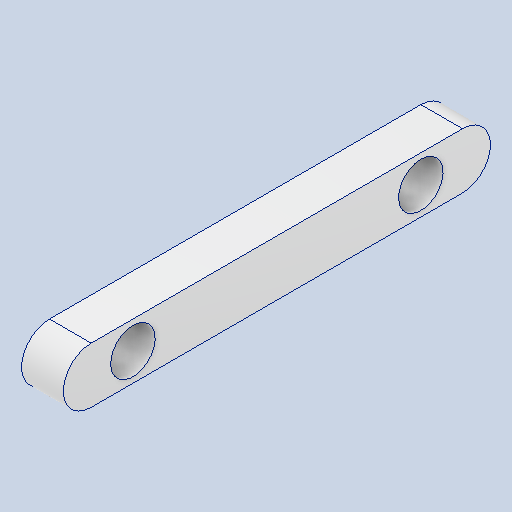
# Autodesk Inventor part: belt_liner_v2_Plate_18
Saved by Autodesk Inventor 2025.2 (Build 292293000, 293)
## iProperties
Created: 2024-12-15
Part Number: belt_liner_v2_Plate_18
Material: アルミニウム 6061
Document SubType Name: Modeling
Designer: haruy
Density: 2.7 g/cm^3
Appearance: アルミニウム - フラット
Author: haruy
Autodesk Inventor part; units mm, degrees
ref_plane "YZ Plane" through (0, 0, 0) normal (1, 0, 0) x (0, 1, 0)
ref_plane "XZ Plane" through (0, 0, 0) normal (0, 1, 0) x (-1, 0, 0)
ref_plane "XY Plane" through (0, 0, 0) normal (0, 0, 1) x (1, 0, 0)
sketch "スケッチ1" plane through (0, 0, 0) normal (1, 0, 0) x (0, 1, 0)
  line L0 (0.8674, 15.35) -> (4.8674, 15.35)
  line L1 (4.8674, 15.35) -> (4.8674, -15.35)
  line L2 (4.8674, -15.35) -> (0.8674, -15.35)
  line L3 (0.8674, -15.35) -> (0.8674, 15.35)
  circle A0 centre (2.8674, 10.35) radius 1.6
  line L4 (0.8674, 9.5) -> (5.8674, 9.5)
  line L5 (5.8674, 9.5) -> (5.8674, -9.5)
  line L6 (5.8674, -9.5) -> (0.8674, -9.5)
  line L7 (0.8674, -9.5) -> (0.8674, 9.5)
  circle A1 centre (2.8674, 10.35) radius 3.5
  line L8 (0.8674, 0) -> (5.8674, 0)
  circle A2 centre (2.8674, -10.35) radius 1.6
  line L9 (0.8674, 9.5) -> (0.3674, 9.5)
  line L10 (0.3674, 9.5) -> (0.3674, -7.3389)
  line L11 (0.3674, -7.3389) -> (0.8674, -7.3389)
  line L12 (0.8674, -7.3389) -> (0.8674, 9.5)
  point P0 (0, 0)
  dimension "d0" = 4
  dimension "d1" = 30.7
  dimension "d2" = 3.2
  dimension "d3" = 5
  dimension "d4" = 19
  dimension "d6" = 5
  dimension "d7" = 2
  dimension "d8" = 7
  dimension "d9" = 0.5
  dimension "d13" = 15.35
  dimension "d14" = 0
  constraints: 26 end point, 6 parallel, 3 centre point, 3 horizontal, 3 perpendicular, 2 midpoint, 1 coincident, 1 point on line, 1 symmetric about line, 1 other
  measures "d0" distance of L1.end L2.end
  measures "d1" distance between parallel lines of L2 L0
  measures "d2" diameter of A0
  measures "d3" distance of L5.end L6.end
  measures "d4" distance of L4.end L5.end
  measures "d6" distance from line of A0.centre L0
  measures "d7" distance from line of A0.centre L3
  measures "d8" diameter of A1
  measures "d9" distance of L11.end L10.end
  measures "d13" distance from line of L0 point (0, 0)
  measures "d14" distance from line of point (0, 0) L8
extrude "押し出し1" add sketch "スケッチ1" along normal blind 3 contours L0 L1 A1 L3 | A1 L1 L4 A0 L3 | L4 A0 L1 A1 L3 | A1 L1 L8 L3 | L8 L1 L6 A2 L3 | L6 A2 L1 L2 L3
fillet "フィレット1" radius 2 4 edges at (1.5, 4.8674, 15.35) (1.5, 0.8674, 15.35) (1.5, 0.8674, -15.35) (1.5, 4.8674, -15.35)
